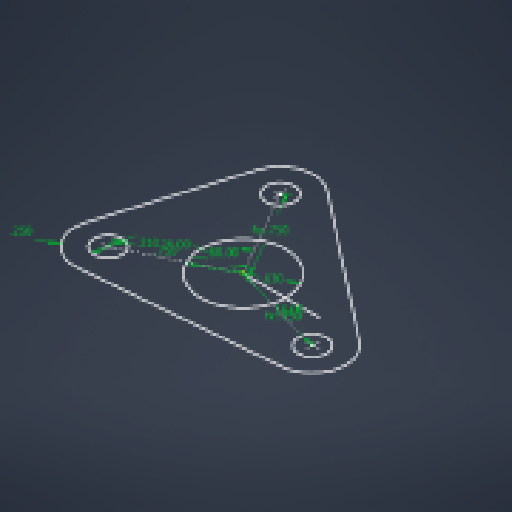
# Autodesk Inventor part: PLATE,BELT,REVERSER
Saved by Autodesk Inventor 2026.1 (Build 301233020, 233B)
## iProperties
Created: 2026-03-30
Part Number: PLATE,BELT,REVERSER
Material: Aluminum 6061
Document SubType Name: Sheet Metal
Designer: Owen L
Density: 2.7 g/cm^3
Sheet Metal Rule: Default
Appearance: Aluminum - Flat
Author: Owen L
Autodesk Inventor part; units mm, degrees
ref_plane "YZ Plane" through (0, 0, 0) normal (1, 0, 0) x (0, 1, 0)
ref_plane "XZ Plane" through (0, 0, 0) normal (0, 1, 0) x (-1, 0, 0)
ref_plane "XY Plane" through (0, 0, 0) normal (0, 0, 1) x (1, 0, 0)
sketch "Sketch1" plane through (0, 0, 0) normal (0, 1, 0) x (-1, 0, 0)
  circle A0 centre (0, 0) radius 11.1125
  line L0 (12.7, -21.997) -> (0, 0) construction
  line L1 (0, 0) -> (22.4269, 11.9246) construction
  line L2 (0, 0) -> (-24.6455, 6.1448) construction
  line L3 (0, 0) -> (-14.4094, 0)
  arc A1 (28.5309, 10.1743) -> (21.653, 18.2272) centre (22.4269, 11.9246) ccw
  arc A2 (8.8785, -27.0684) -> (18.804, -23.7473) centre (12.7, -21.997) ccw
  arc A3 (-25.4194, 12.4475) -> (-28.467, 1.0735) centre (-24.6455, 6.1448) ccw
  line L4 (21.653, 18.2272) -> (-25.4194, 12.4475)
  line L5 (-28.467, 1.0735) -> (8.8785, -27.0684)
  line L6 (18.804, -23.7473) -> (28.5309, 10.1743)
  circle A4 centre (22.4269, 11.9246) radius 2.667
  circle A5 centre (12.7, -21.997) radius 2.667
  circle A6 centre (-24.6455, 6.1448) radius 2.667
  dimension "d0" = 22.225
  dimension "d1" = 25.4
  dimension "d2" = 25.4
  dimension "d3" = 25.4
  dimension "d4" = 14
  dimension "d5" = 28
  dimension "d6" = 60
  dimension "d7" = 6.35
  dimension "d8" = 5.334
  measures "d0" diameter of A0
  measures "d1" distance of L1.end point (0, 0)
  measures "d2" distance of L2.end point (0, 0)
  measures "d3" distance of point (12.7, -21.997) point (0, 0)
  measures "d4" angle of L3 L2
  measures "d5" angle of L3 L1
  measures "d6" angle of L3 L0
  measures "d7" radius of A1
  measures "d8" diameter of A4
extrude "Plate1" add sketch "Sketch1" along normal blind 3.175
equation "\"d9\" = Thickness"
equation "\"d2\" = d1"
equation "\"d3\" = d1"
equation "\"BendRadius\" = Thickness"
equation "\"BendReliefWidth\" = Thickness"
equation "\"BendReliefDepth\" = 0.5 * Thickness"
equation "\"CornerReliefSize\" = 4 * Thickness"
equation "\"MinimumRemnant\" = 2 * Thickness"
equation "\"TransitionRadius\" = BendRadius"
equation "\"JacobiRadiusSize\" = BendRadius"
equation "\"GapSize\" = Thickness"
equation "\"Thickness\" = 3.175"
body "Solid1"
